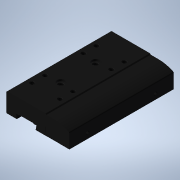
# Autodesk Inventor part: EGC-80-GK-GPTB1--------(0)
Saved by Autodesk Inventor 2021 (Build 250183000, 183)
## iProperties
Created: 2026-04-25
Part Number: EGC-80-GK-GPTB1--------(0)
Material: Generic
Catalog Web Link: www.3dfindit.com
Description: EGC_WAG-Schliten EGC
Vendor: FESTO
Document SubType Name: Modeling
Designer: psAdmin
Manufacturer: FESTO
Mass: 168.578 g
Surface Area: 283.261 cm^2
Volume: 168.578 cm^3
Density: 1 g/cm^3
Appearance: PSOLRGB-128-128-128
Category: PARTsolutions
Company: FESTO
Title: EGC-80-GK-GPTB1--------(0)
Author: Cadenas PARTsolutions
Comments: Schliten EGC
PSOL_IDENT_0: {$CADENAS_DATA/23d-libs/festo/parts/e/egc/parts/egc_wagen.prj},220 {VTYP=3D},{NB=EGC-80-GK-GPTB1----
PSOL_IDENT_1: ----(0)},{LINA=EGC-80-GK-GPTB1--------(0)},{NN=EGC_WAG},{DATE=04.02.2025 22:30:31},{GEOMDATE=04.02.2
PSOL_IDENT_2: 025 22:30:31},{VERSION=},{LINEID=30},{WBVAR=FKT,SL,SA,HGO,ZSL,ZSR},{WBNUMERIC=SL,HGO}  {NB=EGC-80-GK
PSOL_IDENT_3: -GPTB1--------(0)},{LINA=EGC-80-GK-GPTB1--------(0)},{KT=DUMMY},{TYP=EGC-80-GK-GP},{VERS=4},{SIZE=80
PSOL_IDENT_4: },{L=120},{FKT=TB},{SL=1},{SA=-},{HGO=0},{ZSL=-},{ZSR=-}
NB: EGC-80-GK-GPTB1--------(0)
NN: EGC_WAG
NT: Schliten EGC
NBSYN: $TYP.$FKT.$SL.$SA.-$ZSL.-$ZSR.---($HGO.)
LINA: EGC-80-GK-GPTB1--------(0)
CATALOG: Festo
TYP: EGC-80-GK-GP
VERS: 4
SIZE: 80
L: 120
FKT: TB
SL: 1
SA: -
HGO: 0
ZSL: -
ZSR: -
SUPPLIER: FESTO
ARTICLENO: EGC-80-GK-GPTB1--------(0)
BOMINFO: EGC-80-GK-GPTB1--------(0)
CREATOR: CADENAS GmbH
Autodesk Inventor part; units mm, degrees
sketch "Sketch_1" plane through (0, 0, 0) normal (0, 0, 1) x (1, 0, 0)
  line L0 (0, 12) -> (0.2, 12)
  line L1 (0.2, 12) -> (0.2, 0)
  line L2 (0.2, 0) -> (3.5, 0)
  line L3 (3.5, 0) -> (3.5, 11.6)
  line L4 (3.5, 11.6) -> (42.5, 11.6)
  line L5 (42.5, 11.6) -> (42.5, 0)
  line L6 (42.5, 0) -> (72.6, 0)
  line L7 (72.6, 0) -> (72.6, 16.8029)
  arc A0 (72.6, 16.8029) -> (55, 21) centre (55, -18) ccw
  line L8 (55, 21) -> (46, 21)
  line L9 (46, 21) -> (46, 22)
  line L10 (46, 22) -> (0, 22)
  line L11 (0, 22) -> (0, 12)
  constraints: 24 end point, 2 point on circle, 1 centre point
extrude "Extrusion1" add sketch "Sketch_1" against normal blind 120
sketch "Sketch_2" plane through (0, 0, 0) normal (0, 0, 1) x (1, 0, 0)
  line L0 (-5, 27) -> (-5, -5)
  line L1 (-5, -5) -> (85, -5)
  line L2 (85, -5) -> (85, 27)
  line L3 (85, 27) -> (-5, 27)
  line L4 (0, 12) -> (0.2, 12)
  line L5 (0.2, 12) -> (0.2, 1)
  arc A0 (0.2, 1) -> (1.2, 0) centre (1.2, 1) ccw
  line L6 (1.2, 0) -> (72.6, 0)
  line L7 (72.6, 0) -> (72.6, 16.057)
  arc A1 (72.6, 16.057) -> (71.9206, 17.1382) centre (71.4, 16.057) ccw
  arc A2 (71.9206, 17.1382) -> (55, 21) centre (55, -18) ccw
  line L8 (55, 21) -> (46, 21)
  line L9 (46, 21) -> (46, 21.2)
  line L10 (46, 21.2) -> (45.2, 22)
  line L11 (45.2, 22) -> (1, 22)
  line L12 (1, 22) -> (0, 21)
  line L13 (0, 21) -> (0, 12)
  constraints: 28 end point, 6 point on circle, 3 centre point
extrude "Extrusion2" cut sketch "Sketch_2" against normal blind 120
sketch "Sketch_28" plane through (0, 0, -60) normal (0, 0, 1) x (1, 0, 0)
  line L0 (3.5, 11.6) -> (3.5, 0)
  line L1 (3.5, 0) -> (11, 0)
  line L2 (11, 0) -> (11, 5.5)
  line L3 (11, 5.5) -> (35, 5.5)
  line L4 (35, 5.5) -> (35, 0)
  line L5 (35, 0) -> (42.5, 0)
  line L6 (42.5, 0) -> (42.5, 11.6)
  line L7 (42.5, 11.6) -> (3.5, 11.6)
  constraints: 16 end point
extrude "Extrusion3" add sketch "Sketch_28" along normal mid plane 120
sketch "Sketch_3" plane through (0, 0, -60) normal (0, 0, 1) x (1, 0, 0)
  line L0 (3.5, 11.6) -> (3.5, 0)
  line L1 (3.5, 0) -> (12.1883, 0)
  line L2 (12.1883, 0) -> (11.5169, 2.5055)
  arc A0 (11.5169, 2.5055) -> (11, 4.164) centre (10.73, 3.17) ccw
  line L3 (11, 4.164) -> (11, 4.9)
  line L4 (11, 4.9) -> (13.5186, 4.9)
  arc A1 (13.5186, 4.9) -> (15.064, 5.5) centre (14.07, 5.77) ccw
  line L5 (15.064, 5.5) -> (30.936, 5.5)
  arc A2 (30.936, 5.5) -> (32.4814, 4.9) centre (31.93, 5.77) ccw
  line L6 (32.4814, 4.9) -> (35, 4.9)
  line L7 (35, 4.9) -> (35, 4.164)
  arc A3 (35, 4.164) -> (34.4831, 2.5055) centre (35.27, 3.17) ccw
  line L8 (34.4831, 2.5055) -> (33.8117, 0)
  line L9 (33.8117, 0) -> (42.5, 0)
  line L10 (42.5, 0) -> (42.5, 11.6)
  line L11 (42.5, 11.6) -> (3.5, 11.6)
  constraints: 24 end point, 8 point on circle, 4 centre point
extrude "Extrusion4" add sketch "Sketch_3" along normal mid plane 120
sketch "Sketch_20" plane through (0, 0, 0) normal (0, 0, 1) x (1, 0, 0)
  line L0 (45.5, 3) -> (47.875, 3)
  line L1 (47.875, 3) -> (47.875, 0)
  line L2 (47.875, 0) -> (62.125, 0)
  line L3 (62.125, 0) -> (62.125, 3)
  line L4 (62.125, 3) -> (64.5, 3)
  line L5 (64.5, 3) -> (64.5, 9)
  line L6 (64.5, 9) -> (45.5, 9)
  line L7 (45.5, 9) -> (45.5, 3)
  constraints: 16 end point
extrude "Extrusion5" cut sketch "Sketch_20" against normal blind 0.1
sketch "Sketch_21" plane through (0, 0, -120) normal (0, 0, 1) x (1, 0, 0)
  line L0 (45.5, 3) -> (47.875, 3)
  line L1 (47.875, 3) -> (47.875, 0)
  line L2 (47.875, 0) -> (62.125, 0)
  line L3 (62.125, 0) -> (62.125, 3)
  line L4 (62.125, 3) -> (64.5, 3)
  line L5 (64.5, 3) -> (64.5, 9)
  line L6 (64.5, 9) -> (45.5, 9)
  line L7 (45.5, 9) -> (45.5, 3)
  constraints: 16 end point
extrude "Extrusion6" cut sketch "Sketch_21" along normal blind 0.1
sketch "Sketch7" plane through (72.6, 0, 0) normal (1, 0, 0) x (0, 0, -1)
  point P0 (21, 6)
hole "Hole1" at (72.6, 6, -21) direction (-1, 0, 0) diameter 3.242 depth 10 tip angle 120 countersink diameter 4 countersink angle 90 thread size "M4x0.7" class "6H" standard "ISO Metric profile"
sketch "Sketch8" plane through (72.6, 0, 0) normal (1, 0, 0) x (0, 0, -1)
  point P0 (99, 6)
hole "Hole2" at (72.6, 6, -99) direction (-1, 0, 0) diameter 3.242 depth 10 tip angle 120 countersink diameter 4 countersink angle 90 thread size "M4x0.7" class "6H" standard "ISO Metric profile"
sketch "Sketch_8" plane through (7, 0, 0) normal (1, 0, 0) x (0, 0, -1)
  line L0 (23, 14.5) -> (23, 22)
  line L1 (23, 22) -> (25.5, 22)
  line L2 (25.5, 22) -> (25.067, 21.567)
  line L3 (25.067, 21.567) -> (25.067, 14.5)
  line L4 (25.067, 14.5) -> (23, 14.5)
  line L5 (23, 14.5) -> (23, 22)
  constraints: 12 end point
revolve "Revolution1" cut sketch "Sketch_8" angle 360 about axis through (7, 14.5, -23) along (0, -1, 0)
thread "Thread1" size "M5x0.8" class "6H" standard "ISO Metric profile" full length
sketch "Pattern_1_Sketch_8_0" plane through (39, 0, 0) normal (1, 0, 0) x (0, 0, -1)
  line L0 (23, 14.5) -> (23, 22)
  line L1 (23, 22) -> (25.5, 22)
  line L2 (25.5, 22) -> (25.067, 21.567)
  line L3 (25.067, 21.567) -> (25.067, 14.5)
  line L4 (25.067, 14.5) -> (23, 14.5)
  line L5 (23, 14.5) -> (23, 22)
  constraints: 12 end point
revolve "Revolution2" cut sketch "Pattern_1_Sketch_8_0" angle 360 about axis through (39, 14.5, -23) along (0, -1, 0)
thread "Thread2" size "M5x0.8" class "6H" standard "ISO Metric profile" full length
sketch "Pattern_1_Sketch_8_1" plane through (39, 0, 0) normal (1, 0, 0) x (0, 0, -1)
  line L0 (38, 14.5) -> (38, 22)
  line L1 (38, 22) -> (40.5, 22)
  line L2 (40.5, 22) -> (40.067, 21.567)
  line L3 (40.067, 21.567) -> (40.067, 14.5)
  line L4 (40.067, 14.5) -> (38, 14.5)
  line L5 (38, 14.5) -> (38, 22)
  constraints: 12 end point
revolve "Revolution3" cut sketch "Pattern_1_Sketch_8_1" angle 360 about axis through (39, 14.5, -38) along (0, -1, 0)
thread "Thread3" size "M5x0.8" class "6H" standard "ISO Metric profile" full length
sketch "Pattern_1_Sketch_8_2" plane through (7, 0, 0) normal (1, 0, 0) x (0, 0, -1)
  line L0 (38, 14.5) -> (38, 22)
  line L1 (38, 22) -> (40.5, 22)
  line L2 (40.5, 22) -> (40.067, 21.567)
  line L3 (40.067, 21.567) -> (40.067, 14.5)
  line L4 (40.067, 14.5) -> (38, 14.5)
  line L5 (38, 14.5) -> (38, 22)
  constraints: 12 end point
revolve "Revolution4" cut sketch "Pattern_1_Sketch_8_2" angle 360 about axis through (7, 14.5, -38) along (0, -1, 0)
thread "Thread4" size "M5x0.8" class "6H" standard "ISO Metric profile" full length
sketch "Pattern_1_Sketch_8_3" plane through (39, 0, 0) normal (1, 0, 0) x (0, 0, -1)
  line L0 (82, 14.5) -> (82, 22)
  line L1 (82, 22) -> (84.5, 22)
  line L2 (84.5, 22) -> (84.067, 21.567)
  line L3 (84.067, 21.567) -> (84.067, 14.5)
  line L4 (84.067, 14.5) -> (82, 14.5)
  line L5 (82, 14.5) -> (82, 22)
  constraints: 12 end point
revolve "Revolution5" cut sketch "Pattern_1_Sketch_8_3" angle 360 about axis through (39, 14.5, -82) along (0, -1, 0)
thread "Thread5" size "M5x0.8" class "6H" standard "ISO Metric profile" full length
sketch "Pattern_1_Sketch_8_4" plane through (7, 0, 0) normal (1, 0, 0) x (0, 0, -1)
  line L0 (82, 14.5) -> (82, 22)
  line L1 (82, 22) -> (84.5, 22)
  line L2 (84.5, 22) -> (84.067, 21.567)
  line L3 (84.067, 21.567) -> (84.067, 14.5)
  line L4 (84.067, 14.5) -> (82, 14.5)
  line L5 (82, 14.5) -> (82, 22)
  constraints: 12 end point
revolve "Revolution6" cut sketch "Pattern_1_Sketch_8_4" angle 360 about axis through (7, 14.5, -82) along (0, -1, 0)
thread "Thread6" size "M5x0.8" class "6H" standard "ISO Metric profile" full length
sketch "Pattern_1_Sketch_8_5" plane through (39, 0, 0) normal (1, 0, 0) x (0, 0, -1)
  line L0 (97, 14.5) -> (97, 22)
  line L1 (97, 22) -> (99.5, 22)
  line L2 (99.5, 22) -> (99.067, 21.567)
  line L3 (99.067, 21.567) -> (99.067, 14.5)
  line L4 (99.067, 14.5) -> (97, 14.5)
  line L5 (97, 14.5) -> (97, 22)
  constraints: 12 end point
revolve "Revolution7" cut sketch "Pattern_1_Sketch_8_5" angle 360 about axis through (39, 14.5, -97) along (0, -1, 0)
thread "Thread7" size "M5x0.8" class "6H" standard "ISO Metric profile" full length
sketch "Pattern_1_Sketch_8_6" plane through (7, 0, 0) normal (1, 0, 0) x (0, 0, -1)
  line L0 (97, 14.5) -> (97, 22)
  line L1 (97, 22) -> (99.5, 22)
  line L2 (99.5, 22) -> (99.067, 21.567)
  line L3 (99.067, 21.567) -> (99.067, 14.5)
  line L4 (99.067, 14.5) -> (97, 14.5)
  line L5 (97, 14.5) -> (97, 22)
  constraints: 12 end point
revolve "Revolution8" cut sketch "Pattern_1_Sketch_8_6" angle 360 about axis through (7, 14.5, -97) along (0, -1, 0)
thread "Thread8" size "M5x0.8" class "6H" standard "ISO Metric profile" full length
sketch "Sketch_10" plane through (23, 0, 0) normal (1, 0, 0) x (0, 0, -1)
  line L0 (40, 19.9) -> (40, 13.4)
  line L1 (40, 13.4) -> (37.5415, 13.4)
  line L2 (37.5415, 13.4) -> (37.5415, 19.3585)
  line L3 (37.5415, 19.3585) -> (37, 19.9)
  line L4 (37, 19.9) -> (35.5, 19.9)
  line L5 (35.5, 19.9) -> (35.5, 22)
  line L6 (35.5, 22) -> (40, 22)
  line L7 (40, 22) -> (40, 13.4)
  constraints: 16 end point
revolve "Revolution9" cut sketch "Sketch_10" angle 360 about axis through (23, 19.9, -40) along (0, 1, 0)
thread "Thread9" size "M6x1" class "6H" standard "ISO Metric profile" full length
sketch "Sketch_11" plane through (23, 0, 0) normal (1, 0, 0) x (0, 0, -1)
  line L0 (80, 19.9) -> (80, 13.4)
  line L1 (80, 13.4) -> (77.5415, 13.4)
  line L2 (77.5415, 13.4) -> (77.5415, 19.3585)
  line L3 (77.5415, 19.3585) -> (77, 19.9)
  line L4 (77, 19.9) -> (75.5, 19.9)
  line L5 (75.5, 19.9) -> (75.5, 22)
  line L6 (75.5, 22) -> (80, 22)
  line L7 (80, 22) -> (80, 13.4)
  constraints: 16 end point
revolve "Revolution10" cut sketch "Sketch_11" angle 360 about axis through (23, 19.9, -80) along (0, 1, 0)
thread "Thread10" size "M6x1" class "6H" standard "ISO Metric profile" full length
sketch "Sketch27" plane through (0, 12, -120) normal (-1, 0, 0) x (0, 0, 1)
  point P0 (75, 5)
hole "Hole3" at (0, 17, -45) direction (1, 0, 0) diameter 4.134 depth 14 tip angle 120 countersink diameter 5 countersink angle 90 thread size "M5x0.8" class "6H" standard "ISO Metric profile"
sketch "Sketch28" plane through (0, 12, -120) normal (-1, 0, 0) x (0, 0, 1)
  point P0 (45, 5)
hole "Hole4" at (0, 17, -75) direction (1, 0, 0) diameter 4.134 depth 14 tip angle 120 countersink diameter 5 countersink angle 90 thread size "M5x0.8" class "6H" standard "ISO Metric profile"
sketch "Sketch_14" plane through (0, 17, 0) normal (0, 1, 0) x (1, 0, 0)
  line L0 (2.1, 30) -> (0, 30)
  line L1 (0, 30) -> (0, 33.5)
  line L2 (0, 33.5) -> (2.1, 33.5)
  line L3 (2.1, 33.5) -> (2.1, 30)
  line L4 (2.1, 30) -> (0, 30)
  constraints: 10 end point
revolve "Revolution11" cut sketch "Sketch_14" angle 360 about axis through (2.1, 17, -30) along (1, 0, 0)
sketch "Sketch_15" plane through (0, 17, 0) normal (0, 1, 0) x (1, 0, 0)
  line L0 (2.1, 90) -> (0, 90)
  line L1 (0, 90) -> (0, 93.5)
  line L2 (0, 93.5) -> (2.1, 93.5)
  line L3 (2.1, 93.5) -> (2.1, 90)
  line L4 (2.1, 90) -> (0, 90)
  constraints: 10 end point
revolve "Revolution12" cut sketch "Sketch_15" angle 360 about axis through (2.1, 17, -90) along (1, 0, 0)
ref_plane "1NPN_XY" through (23, 22, -60) normal (0, 1, 0) x (1, 0, 0)
ref_plane "1NPN_YZ" through (23, 22, -60) normal (1, 0, 0) x (0, 0, -1)
ref_plane "1NPN_ZX" through (23, 22, -60) normal (0, 0, -1) x (0, 1, 0)
ref_plane "BP1_1_XY" through (3.5, 13.5, 6.5) normal (1, 0, 0) x (0, 0, -1)
ref_plane "BP1_1_YZ" through (3.5, 13.5, 6.5) normal (0, 0, -1) x (0, 1, 0)
ref_plane "BP1_1_ZX" through (3.5, 13.5, 6.5) normal (0, 1, 0) x (1, 0, 0)
ref_plane "BP1_2_XY" through (3.5, 13.5, -126.5) normal (1, 0, 0) x (0, 0, -1)
ref_plane "BP1_2_YZ" through (3.5, 13.5, -126.5) normal (0, 0, -1) x (0, 1, 0)
ref_plane "BP1_2_ZX" through (3.5, 13.5, -126.5) normal (0, 1, 0) x (1, 0, 0)
ref_plane "BP2_1_XY" through (42.5, 13.5, 6.5) normal (1, 0, 0) x (0, 0, -1)
ref_plane "BP2_1_YZ" through (42.5, 13.5, 6.5) normal (0, 0, -1) x (0, 1, 0)
ref_plane "BP2_1_ZX" through (42.5, 13.5, 6.5) normal (0, 1, 0) x (1, 0, 0)
ref_plane "BP2_2_XY" through (42.5, 13.5, -126.5) normal (1, 0, 0) x (0, 0, -1)
ref_plane "BP2_2_YZ" through (42.5, 13.5, -126.5) normal (0, 0, -1) x (0, 1, 0)
ref_plane "BP2_2_ZX" through (42.5, 13.5, -126.5) normal (0, 1, 0) x (1, 0, 0)
ref_plane "BP3_XY" through (23, 21, 6.5) normal (0, 1, 0) x (1, 0, 0)
ref_plane "BP3_YZ" through (23, 21, 6.5) normal (1, 0, 0) x (0, 0, -1)
ref_plane "BP3_ZX" through (23, 21, 6.5) normal (0, 0, -1) x (0, 1, 0)
ref_plane "BP5_XY" through (23, 21, -126.5) normal (0, 1, 0) x (1, 0, 0)
ref_plane "BP5_YZ" through (23, 21, -126.5) normal (1, 0, 0) x (0, 0, -1)
ref_plane "BP5_ZX" through (23, 21, -126.5) normal (0, 0, -1) x (0, 1, 0)
ref_plane "EXPT_BLOCK_XY" through (23, 22, -40) normal (0, -1, 0) x (1, 0, 0)
ref_plane "EXPT_BLOCK_YZ" through (23, 22, -40) normal (1, 0, 0) x (0, 0, 1)
ref_plane "EXPT_BLOCK_ZX" through (23, 22, -40) normal (0, 0, 1) x (0, -1, 0)
ref_plane "EXPT_HALTEWINKEL_H_XY" through (0, 17, -60) normal (1, 0, 0) x (0, 0, -1)
ref_plane "EXPT_HALTEWINKEL_H_YZ" through (0, 17, -60) normal (0, 0, -1) x (0, 1, 0)
ref_plane "EXPT_HALTEWINKEL_H_ZX" through (0, 17, -60) normal (0, 1, 0) x (1, 0, 0)
ref_plane "EXPT_HALTEWINKEL_V_XY" through (72.6, 6, -60) normal (-1, 0, 0) x (0, 0, -1)
ref_plane "EXPT_HALTEWINKEL_V_YZ" through (72.6, 6, -60) normal (0, 0, -1) x (0, -1, 0)
ref_plane "EXPT_HALTEWINKEL_V_ZX" through (72.6, 6, -60) normal (0, -1, 0) x (-1, 0, 0)
ref_plane "SCHALTFAHNE_XY" through (72.6, 6, -60) normal (-1, 0, 0) x (0, 0, -1)
ref_plane "SCHALTFAHNE_YZ" through (72.6, 6, -60) normal (0, 0, -1) x (0, -1, 0)
ref_plane "SCHALTFAHNE_ZX" through (72.6, 6, -60) normal (0, -1, 0) x (-1, 0, 0)
ref_plane "SCHLITTEN_XY" through (23, -1.5, -60) normal (0, 0, -1) x (1, 0, 0)
ref_plane "SCHLITTEN_YZ" through (23, -1.5, -60) normal (1, 0, 0) x (0, -1, 0)
ref_plane "SCHLITTEN_ZX" through (23, -1.5, -60) normal (0, -1, 0) x (0, 0, -1)
ref_plane "SENSOR_XY" through (0, 17, -75) normal (1, 0, 0) x (0, 0, -1)
ref_plane "SENSOR_YZ" through (0, 17, -75) normal (0, 0, -1) x (0, 1, 0)
ref_plane "SENSOR_ZX" through (0, 17, -75) normal (0, 1, 0) x (1, 0, 0)
body "Solid1"
